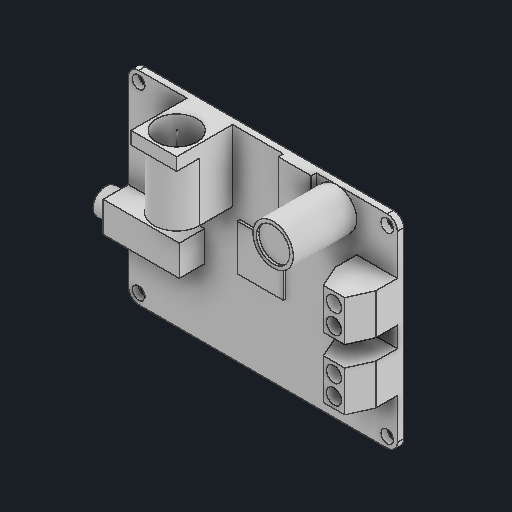
# Autodesk Inventor part: Max9744_20W_ClassD_Amplifier
Saved by Autodesk Inventor 2025.2 (Build 292293000, 293)
## iProperties
Created: 2025-09-18
Part Number: Max9744_20W_ClassD_Amplifier
Material: Generic
Document SubType Name: Modeling
Designer: valer
Density: 1 g/cm^3
Appearance: Default
Author: valer
Autodesk Inventor part; units mm, degrees
ref_plane "YZ Plane" through (0, 0, 0) normal (1, 0, 0) x (0, 1, 0)
ref_plane "XZ Plane" through (0, 0, 0) normal (0, 1, 0) x (-1, 0, 0)
ref_plane "XY Plane" through (0, 0, 0) normal (0, 0, 1) x (1, 0, 0)
sketch "Base" plane through (0, 0, 0) normal (0, 0, 1) x (1, 0, 0)
  line L0 (26.5, -20) -> (-26.5, -20)
  line L1 (-26.5, -20) -> (-26.5, 20)
  line L2 (-26.5, 20) -> (26.5, 20)
  line L3 (26.5, 20) -> (26.5, -20)
  line L4 (26.5, -20) -> (-26.5, 20) construction
  line L5 (-26.5, -20) -> (26.5, 20) construction
  point P0 (0, 0)
  dimension "d0" = 53
  dimension "d1" = 40
  constraints: 12 end point, 2 midpoint, 2 parallel, 1 horizontal, 1 perpendicular
  measures "d0" distance of L1.end L2.end
  measures "d1" distance of L0.end L1.end
extrude "BaseFeature" add sketch "Base" along normal blind 1.25
fillet "BaseFilletFeature" radius 2 4 edges at (-26.5, 20, 0.625) (26.5, 20, 0.625) (-26.5, -20, 0.625) (26.5, -20, 0.625)
sketch "MountHoles" plane through (0, 0, 1.25) normal (0, 0, 1) x (1, 0, 0)
  arc A0 (-24.5, 20) -> (-26.5, 18) centre (-24.5, 18) ccw projected
  arc A1 (26.5, 18) -> (24.5, 20) centre (24.5, 18) ccw projected
  arc A2 (-26.5, -18) -> (-24.5, -20) centre (-24.5, -18) ccw projected
  arc A3 (24.5, -20) -> (26.5, -18) centre (24.5, -18) ccw projected
  circle A4 centre (-24.5, 18) radius 1.25
  circle A5 centre (24.5, 18) radius 1.25
  circle A6 centre (-24.5, -18) radius 1.25
  circle A7 centre (24.5, -18) radius 1.25
  point P0 (0, 0)
  dimension "d5" = 2.5
  constraints: 4 centre point, 4 coincident, 3 equal radius
  measures "d5" diameter of A4
extrude "MountHolesFeature" cut sketch "MountHoles" against normal through all
sketch "Sketch3" plane through (0, 0, 1.25) normal (0, 0, 1) x (1, 0, 0)
  line L0 (26.5, 10) -> (18.5, 10)
  line L1 (18.5, 10) -> (18.5, 2)
  line L2 (18.5, 2) -> (26.5, 2)
  line L3 (26.5, 2) -> (26.5, 10)
  line L4 (26.5, -2) -> (18.5, -2)
  line L5 (18.5, -2) -> (18.5, -10)
  line L6 (18.5, -10) -> (26.5, -10)
  line L7 (26.5, -10) -> (26.5, -2)
  line L8 (24.5, 20) -> (-24.5, 20) projected
  line L9 (-24.5, -20) -> (24.5, -20) projected
  line L10 (26.5, -18) -> (26.5, 18) projected
  point P0 (0, 0)
  point P1 (22.5, 10)
  dimension "d8" = 10
  dimension "d9" = 8
  dimension "d10" = 10
  dimension "d11" = 8
  constraints: 16 end point, 4 parallel, 2 collinear, 2 horizontal, 2 perpendicular, 2 point on line, 1 midpoint
  measures "d8" distance from line of point (22.5, 10) L8
  measures "d9" distance of L2.end L0.start
  measures "d10" distance between parallel lines of L6 L9
  measures "d11" distance of L0.start L0.end
extrude "Extrusion3" add sketch "Sketch3" along normal blind 8.5
sketch "Sketch4" plane through (18.5, -10, 1.25) normal (0, -1, 0) x (1, 0, 0)
  line L0 (0, 0) -> (0, 8.5) projected
  line L1 (0, 4.25) -> (8, 4.25)
  line L2 (8, 0) -> (8, 8.5) projected
  line L3 (0, 4.25) -> (1.8922, 8.5)
  line L4 (0, 8.5) -> (8, 8.5) projected
  line L5 (8, 4.25) -> (6.1078, 8.5)
  point P0 (-18.5, -1.25)
  dimension "d14" = 24
  dimension "d15" = 24
  constraints: 6 end point, 2 midpoint, 2 point on line
  measures "d14" angle of L3 L0
  measures "d15" angle of L2 L5
extrude "Extrusion4" cut sketch "Sketch4" along normal through all both and the other way through all contours L0 L4 L3 | L5 L4 L2
sketch "Sketch5" plane through (0, 0, 9.75) normal (0, 0, 1) x (1, 0, 0)
  line L0 (20.3922, 10) -> (20.3922, 2) construction
  line L1 (20.3922, 6) -> (24.6078, 6) construction
  line L2 (24.6078, 2) -> (24.6078, 10) construction
  circle A0 centre (22.5, 7.8922) radius 2.1078 construction
  line L3 (24.6078, 10) -> (20.3922, 10) construction
  circle A1 centre (22.5, 4.1078) radius 2.1078 construction
  line L4 (20.3922, 2) -> (24.6078, 2) construction
  circle A2 centre (22.5, 7.8922) radius 1.5
  circle A3 centre (22.5, 4.1078) radius 1.5
  point P0 (0, 0)
  dimension "d18" = 3
  dimension "d19" = 3
  constraints: 6 tangent, 4 centre point, 2 coincident, 2 end point, 2 midpoint
  measures "d18" diameter of A2
  measures "d19" diameter of A3
extrude "Extrusion5" cut sketch "Sketch5" against normal blind 4
mirror "Mirror1" about plane through (0, 0, 0) normal (0, 1, 0) of "Extrusion5"
sketch "Sketch6" plane through (0, 0, 1.25) normal (0, 0, 1) x (1, 0, 0)
  circle A0 centre (14.5, 16) radius 4
  line L0 (24.5, 20) -> (-24.5, 20) projected
  line L1 (10.5, 20) -> (18.5, 20)
  line L2 (18.5, 20) -> (18.5, 12) construction
  line L3 (18.5, 12) -> (10.5, 12) construction
  line L4 (10.5, 12) -> (10.5, 20) construction
  line L5 (26.5, 10) -> (26.5, 18) projected
  point P0 (0, 0)
  dimension "d22" = 8
  dimension "d23" = 8
  constraints: 8 end point, 4 tangent, 2 parallel, 1 centre point, 1 horizontal, 1 perpendicular, 1 point on line
  measures "d22" diameter of A0
  measures "d23" distance between parallel lines of L5 L2
extrude "Extrusion6" add sketch "Sketch6" along normal blind 12.5
sketch "Sketch7" plane through (14.5, 16, 13.75) normal (0, 0, 1) x (1, 0, 0)
  circle A0 centre (0, 0) radius 4 projected
  circle A1 centre (0, 0) radius 3.3
  point P0 (-14.5, -16)
  dimension "d26" = 0.7
  constraints: 1 centre point, 1 coincident
  measures "d26" radial gap between concentric circles of A0 A1
extrude "Extrusion7" cut sketch "Sketch7" against normal blind 0.5 contours A1
sketch "Sketch8" plane through (0, 0, 1.25) normal (0, 0, 1) x (1, 0, 0)
  line L0 (-26.5, 18) -> (-26.5, -18) projected
  line L1 (-26.5, -0.5) -> (-11.5, -0.5)
  line L2 (-11.5, -0.5) -> (-11.5, -6.5)
  line L3 (-11.5, -6.5) -> (-26.5, -6.5)
  line L4 (-26.5, -6.5) -> (-26.5, -0.5)
  line L5 (-24.5, -20) -> (24.5, -20) projected
  point P0 (0, 0)
  dimension "d29" = 15
  dimension "d30" = 6
  dimension "d31" = 13.5
  constraints: 8 end point, 2 parallel, 1 horizontal, 1 perpendicular, 1 point on line
  measures "d29" distance of L1.start L1.end
  measures "d30" distance of L1.end L2.end
  measures "d31" distance between parallel lines of L5 L3
extrude "Extrusion8" add sketch "Sketch8" along normal blind 5
sketch "Sketch9" plane through (-26.5, -18, 0) normal (-1, 0, 0) x (0, 0, 1)
  line L0 (1.25, 17.5) -> (6.25, 17.5) construction
  line L1 (6.25, 17.5) -> (6.25, 11.5) construction
  line L2 (1.25, 11.5) -> (6.25, 11.5) construction
  circle A0 centre (3.25, 14.5) radius 3 construction
  circle A1 centre (3.25, 14.5) radius 2.5
  circle A2 centre (3.25, 14.5) radius 2
  point P0 (0, 18)
  dimension "d34" = 0.5
  dimension "d35" = 0.5
  constraints: 3 centre point, 3 tangent, 2 coincident
  measures "d34" radial gap between concentric circles of A0 A1
  measures "d35" radial gap between concentric circles of A1 A2
extrude "Extrusion9" add sketch "Sketch9" along normal blind 2.5
sketch "Sketch10" plane through (0, 0, 1.25) normal (0, 0, 1) x (1, 0, 0)
  line L0 (14.5, 20) -> (-24.5, 20) projected
  line L1 (-15, 20) -> (-6, 20)
  line L2 (-6, 20) -> (-6, 6)
  line L3 (-6, 6) -> (-15, 6)
  line L4 (-15, 6) -> (-15, 20)
  line L5 (-26.5, 18) -> (-26.5, -0.5) projected
  point P0 (0, 0)
  dimension "d38" = 14
  dimension "d39" = 9
  dimension "d40" = 11.5
  constraints: 8 end point, 2 parallel, 1 horizontal, 1 perpendicular, 1 point on line
  measures "d38" distance of L3.end L1.start
  measures "d39" distance of L2.end L3.end
  measures "d40" distance between parallel lines of L5 L4
extrude "Extrusion10" add sketch "Sketch10" along normal blind 11
sketch "Sketch11" plane through (-24.5, 20, 0) normal (0, 1, 0) x (1, 0, 0)
  line L0 (18.5, -1.25) -> (18.5, -12.25) construction
  line L1 (18.5, -12.25) -> (9.5, -12.25) construction
  line L2 (9.5, -1.25) -> (9.5, -12.25) construction
  circle A0 centre (14, -7.75) radius 4.5
  circle A1 centre (14, -7.75) radius 4
  circle A2 centre (14, -7.75) radius 0.125
  point P0 (24.5, 0)
  dimension "d43" = 0.5
  dimension "d44" = 0.25
  constraints: 3 centre point, 3 tangent, 2 coincident
  measures "d43" radial gap between concentric circles of A0 A1
  measures "d44" diameter of A2
extrude "Extrusion11" cut sketch "Sketch11" against normal blind 11 contours A1
sketch "Sketch12" plane through (0, 0, 1.25) normal (0, 0, 1) x (1, 0, 0)
  line L0 (-4.5, -4.5) -> (4.5, -4.5)
  line L1 (4.5, -4.5) -> (4.5, 4.5)
  line L2 (4.5, 4.5) -> (-4.5, 4.5)
  line L3 (-4.5, 4.5) -> (-4.5, -4.5)
  line L4 (-4.5, -4.5) -> (4.5, 4.5) construction
  line L5 (4.5, -4.5) -> (-4.5, 4.5) construction
  point P0 (0, 0)
  dimension "d47" = 9
  constraints: 12 end point, 2 midpoint, 2 parallel, 2 perpendicular, 1 horizontal
  measures "d47" distance of L1.end L2.end
extrude "Extrusion12" add sketch "Sketch12" along normal blind 0.5
sketch "Sketch13" plane through (-15, 6, 1.25) normal (0, -1, 0) x (1, 0, 0)
  circle A0 centre (4.5, 6.5) radius 4 projected
  circle A1 centre (4.5, 6.5) radius 4.5
  line L0 (9, 0) -> (0, 0) projected
  line L1 (9, 0) -> (9, 11) projected
  line L2 (0, 11) -> (9, 11) projected
  line L3 (0, 0) -> (0, 11) projected
  point P0 (15, -1.25)
  point P1 (0, 6.5)
  point P2 (4.5, 11)
  point P3 (9, 6.5)
  constraints: 1 centre point, 1 coincident
extrude "Extrusion13" cut sketch "Sketch13" against normal blind 11.5 contours A1 L2 L1 | A1 L3 L2
sketch "Sketch14" plane through (0, 0, 1.25) normal (0, 0, 1) x (1, 0, 0)
  line L0 (14.5, 20) -> (-6, 20) projected
  line L1 (10.5, 20) -> (4, 20)
  line L2 (4, 20) -> (4, 10.5)
  line L3 (4, 10.5) -> (10.5, 10.5)
  line L4 (10.5, 10.5) -> (10.5, 20)
  circle A0 centre (14.5, 16) radius 4 projected
  point P0 (0, 0)
  point P1 (4, 20)
  dimension "d52" = 6.5
  dimension "d53" = 9.5
  constraints: 8 end point, 2 parallel, 1 horizontal, 1 perpendicular, 1 point on line, 1 vertical, 1 vertical alignment
  measures "d52" distance of L2.end L3.end
  measures "d53" distance of L1.end L2.end
extrude "Extrusion14" add sketch "Sketch14" along normal blind 1 contours L4 L3 L2 L0
sketch "Sketch15" plane through (0, 0, 0) normal (0, 0, -1) x (-1, 0, 0)
  line L0 (26.5, -6.5) -> (26.5, -18) projected
  line L1 (26.5, -3.5) -> (17, -3.5)
  line L2 (17, -3.5) -> (17, -13)
  line L3 (17, -13) -> (26.5, -13)
  line L4 (26.5, -13) -> (26.5, -3.5)
  line L5 (24.5, -20) -> (-24.5, -20) projected
  point P0 (0, 0)
  dimension "d56" = 9.5
  dimension "d57" = 7
  constraints: 8 end point, 2 parallel, 2 perpendicular, 1 horizontal, 1 point on line
  measures "d56" distance of L1.end L2.end
  measures "d57" distance between parallel lines of L5 L3
extrude "Extrusion15" add sketch "Sketch15" along normal blind 5
sketch "Sketch16" plane through (0, 0, -5) normal (0, 0, -1) x (-1, 0, 0)
  line L0 (17, -13) -> (26.5, -13) projected
  line L1 (26.5, -13) -> (26.5, -3.5) projected
  line L2 (26.5, -3.5) -> (17, -3.5) projected
  line L3 (17, -3.5) -> (17, -13) projected
  circle A0 centre (21.75, -8.25) radius 4.75
  point P0 (0, 0)
  constraints: 3 tangent, 1 centre point
extrude "Extrusion16" add sketch "Sketch16" along normal blind 6 draft -2 contours A0
body "Solid1"
